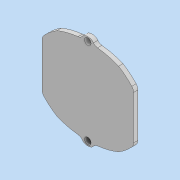
# Autodesk Inventor part: support-miroir
Saved by Autodesk Inventor 2022 (Build 260153000, 153)
## iProperties
Created: 2022-07-29
Part Number: support-miroir
Material: Générique
Document SubType Name: Modeling
Designer: andre
Density: 1 g/cm^3
Appearance: Par défaut
Author: andre
Autodesk Inventor part; units mm, degrees
ref_plane "YZ Plane" through (0, 0, 0) normal (1, 0, 0) x (0, 1, 0)
ref_plane "XZ Plane" through (0, 0, 0) normal (0, 1, 0) x (-1, 0, 0)
ref_plane "XY Plane" through (0, 0, 0) normal (0, 0, 1) x (1, 0, 0)
sketch "Esquisse1" plane through (0, 0, 0) normal (0, 0, 1) x (1, 0, 0)
  ellipse E0 centre (-10.6066, 0) end of major axis (-38.5373, 0) minor radius 19.75 (-15.0725, 19.4959) -> (-24.7487, 17.0312) ccw projected
  ellipse E1 centre (-15.4634, 21.2024) end of major axis (-17.9082, 21.2024) minor radius 1.7287 (-15.0725, 19.4959) -> (-13.2116, 20.529) ccw projected
  ellipse E2 centre (-10.6066, 19.75) end of major axis (-7.7782, 19.75) minor radius 2 (-8.0016, 20.529) -> (-13.2116, 20.529) ccw projected
  ellipse E3 centre (-5.7498, 21.2024) end of major axis (-3.305, 21.2024) minor radius 1.7287 (-8.0016, 20.529) -> (-6.1407, 19.4959) ccw projected
  ellipse E4 centre (-10.6066, 0) end of major axis (17.3241, 0) minor radius 19.75 (3.5355, 17.0312) -> (-6.1407, 19.4959) ccw projected
  ellipse E5 centre (-10.6066, 0) end of major axis (-38.5373, 0) minor radius 19.75 (-24.7487, -17.0312) -> (-15.0725, -19.4959) ccw projected
  ellipse E6 centre (-15.4634, -21.2024) end of major axis (-17.9082, -21.2024) minor radius 1.7287 (-13.2116, -20.529) -> (-15.0725, -19.4959) ccw projected
  ellipse E7 centre (-10.6066, -19.75) end of major axis (-13.435, -19.75) minor radius 2 (-13.2116, -20.529) -> (-8.0016, -20.529) ccw projected
  ellipse E8 centre (-5.7498, -21.2024) end of major axis (-3.305, -21.2024) minor radius 1.7287 (-6.1407, -19.4959) -> (-8.0016, -20.529) ccw projected
  ellipse E9 centre (-10.6066, 0) end of major axis (17.3241, 0) minor radius 19.75 (-6.1407, -19.4959) -> (3.5355, -17.0312) ccw projected
  line L0 (7.3934, 13) -> (-28.6066, 13) construction
  line L1 (-28.6066, 13) -> (-28.6066, -13) construction
  line L2 (-28.6066, -13) -> (7.3934, -13) construction
  line L3 (7.3934, -13) -> (7.3934, 13) construction
  line L4 (7.3934, 13) -> (-28.6066, -13) construction
  line L5 (-28.6066, 13) -> (7.3934, -13) construction
  arc A0 (-31.6066, -11.1719) -> (-24.7487, -17.0312) centre (-9.517, 7.7394) ccw
  line L6 (-31.6066, -11.1719) -> (-31.6066, 0)
  line L7 (-10.6066, 0) -> (-8.2165, 0)
  line L8 (-10.6066, 0) -> (-10.6066, -5.4794)
  arc A1 (-24.7487, 17.0312) -> (-31.6066, 11.1719) centre (-9.517, -7.7394) ccw
  line L9 (-31.6066, 11.1719) -> (-31.6066, 0)
  arc A2 (3.5355, -17.0312) -> (10.3934, -11.1719) centre (-11.6962, 7.7394) ccw
  line L10 (10.3934, -11.1719) -> (10.3934, 0)
  arc A3 (10.3934, 11.1719) -> (3.5355, 17.0312) centre (-11.6962, -7.7394) ccw
  line L11 (10.3934, 11.1719) -> (10.3934, 0)
  point P0 (0, 0)
  point P1 (4.4659, -19.4959)
  point P2 (-4.4659, -19.4959)
  point P3 (14.1421, -17.0312)
  point P4 (14.1421, 17.0312)
  point P5 (-14.1421, -17.0312)
  point P6 (21, 6.606)
  point P7 (14.1424, -17.0311)
  point P8 (14.1419, 17.0313)
  point P9 (0, 19.0996)
  point P10 (-6.6399, 19.0242)
  point P11 (-7.0711, 19.1066)
  point P12 (-14.1418, 17.0314)
  point P13 (21, -6.606)
  dimension "d0" = 36
  dimension "d1" = 26
  dimension "d2" = 29.079
  dimension "d3" = 3
  constraints: 24 end point, 8 point on circle, 7 symmetric about line, 4 centre point, 2 horizontal, 2 midpoint, 2 parallel, 2 perpendicular, 1 point on line, 1 vertical, 14 other
  measures "d0" distance of L1.end L2.end
  measures "d1" distance of L2.end L0.start
  measures "d2" radius of A0
  measures "d3" distance between parallel lines of L1 L6
extrude "Extrusion1" add sketch "Esquisse1" along normal blind 2
fillet "Congé1" radius 3 4 edges at (-31.6066, 11.1719, 1) (-31.6066, -11.1719, 1) (10.3934, 11.1719, 1) (10.3934, -11.1719, 1)
sketch "Esquisse4" plane through (0, 0, 0) normal (0, 0, -1) x (-1, 0, 0)
  ellipse E0 centre (10.6066, 19.75) end of major axis (7.7782, 19.75) minor radius 2 (13.2116, 20.529) -> (8.0016, 20.529) ccw projected
  circle A0 centre (10.6066, 19.75) radius 1.5
  line L0 (0, 0) -> (14.2006, 0)
  circle A1 centre (10.6066, -19.75) radius 1.5
  dimension "d7" = 3
  constraints: 2 centre point, 2 end point, 1 coincident, 1 horizontal, 1 symmetric about line, 2 other
  measures "d7" diameter of A0
extrude "Extrusion2" cut sketch "Esquisse4" against normal up to surface (2 mm away)
